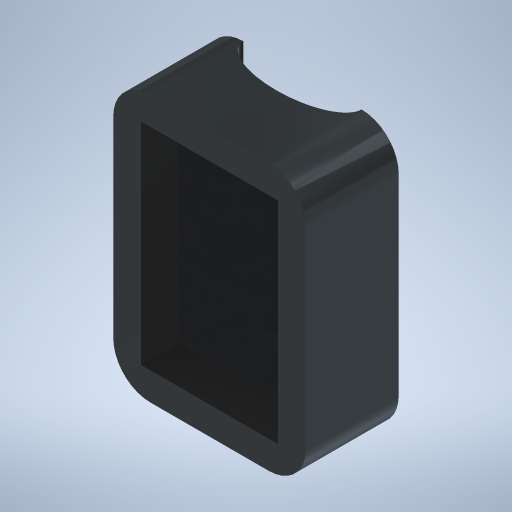
# Autodesk Inventor part: bateria pat 1
Saved by Autodesk Inventor 2023 (Build 270158000, 158)
## iProperties
Created: 2022-10-07
Part Number: bateria pat 1
Material: Generic
Document SubType Name: Modeling
Designer: Xiaba
Density: 1 g/cm^3
Appearance: Polished Diamond Plate
Author: Xiaba
Autodesk Inventor part; units mm, degrees
ref_plane "YZ Plane" through (0, 0, 0) normal (1, 0, 0) x (0, 1, 0)
ref_plane "XZ Plane" through (0, 0, 0) normal (0, 1, 0) x (-1, 0, 0)
ref_plane "XY Plane" through (0, 0, 0) normal (0, 0, 1) x (1, 0, 0)
sketch "Sketch1" plane through (0, 0, 0) normal (0, 0, 1) x (1, 0, 0)
  line L0 (0, 0) -> (-10.3721, 0)
  line L1 (-10.3721, 0) -> (-10.3721, 14.357)
  line L2 (-10.3721, 14.357) -> (0, 14.357)
  line L3 (0, 14.357) -> (0, 0)
  constraints: 8 end point, 2 parallel, 1 horizontal, 1 perpendicular
extrude "Extrusion1" add sketch "Sketch1" along normal blind 5
sketch "Sketch2" plane through (0, 0, 5) normal (0, 0, 1) x (1, 0, 0)
  line L0 (-8.8721, 12.857) -> (-1.5, 12.857)
  line L1 (-1.5, 12.857) -> (-1.5, 1.5)
  line L2 (-1.5, 1.5) -> (-8.8721, 1.5)
  line L3 (-8.8721, 1.5) -> (-8.8721, 12.857)
  line L4 (0, 14.357) -> (-10.3721, 14.357) projected
  line L5 (-10.3721, 0) -> (0, 0) projected
  line L6 (0, 0) -> (0, 14.357) projected
  line L7 (-10.3721, 14.357) -> (-10.3721, 0) projected
  dimension "d2" = 1.5
  dimension "d3" = 1.5
  dimension "d4" = 1.5
  dimension "d5" = 1.5
  constraints: 8 end point, 2 parallel, 1 horizontal, 1 perpendicular
  measures "d2" distance between parallel lines of L0 L4
  measures "d3" distance between parallel lines of L5 L2
  measures "d4" distance between parallel lines of L6 L1
  measures "d5" distance between parallel lines of L7 L3
extrude "Extrusion2" cut sketch "Sketch2" against normal blind 2 contours L0 L1 L2 L3
sketch "Sketch3" plane through (0, 0, 3) normal (0, 0, 1) x (1, 0, 0)
  line L0 (-8.8721, 12.857) -> (-1.5, 12.857) projected
  line L1 (-8.8721, 1.5) -> (-8.8721, 12.857) projected
  line L2 (-1.5, 12.857) -> (-1.5, 1.5) projected
  line L3 (-1.5, 1.5) -> (-8.8721, 1.5) projected
  point P0 (0, 0)
fillet "Fillet1" radius 2 1 edges at (-10.3721, 14.357, 2.5)
fillet "Fillet2" radius 2 1 edges at (0, 14.357, 2.5)
fillet "Fillet3" radius 2 1 edges at (-10.3721, 0, 2.5)
fillet "Fillet4" radius 2 1 edges at (0, 0, 2.5)
sketch "Sketch4" plane through (-8.3721, 0, 0) normal (0, -1, 0) x (1, 0, 0)
  line L0 (6.3721, 0) -> (0, 0) projected
  ellipse E0 centre (3.186, 0) end of major axis (6.3721, 0) minor radius 1.4038
  point P0 (8.3721, 0)
  constraints: 1 horizontal, 1 horizontal alignment, 1 midpoint, 2 other
extrude "Extrusion3" cut sketch "Sketch4" against normal blind 50
body "Solid1"
